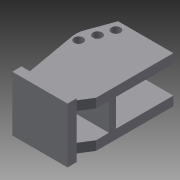
# Autodesk Inventor part: BADAN 3
Saved by Autodesk Inventor 2014 SP2 (Build 180246200, 246)
## iProperties
Created: 2019-06-24
Part Number: BADAN 3
Material: Generic
Document SubType Name: Modeling
Designer: USER PC
Density: 1 g/cm^3
Appearance: Default
Author: USER PC
Autodesk Inventor part; units mm, degrees
ref_plane "YZ Plane" through (0, 0, 0) normal (1, 0, 0) x (0, 1, 0)
ref_plane "XZ Plane" through (0, 0, 0) normal (0, 1, 0) x (-1, 0, 0)
ref_plane "XY Plane" through (0, 0, 0) normal (0, 0, 1) x (1, 0, 0)
sketch "Sketch1" plane through (0, 0, 0) normal (0, 0, 1) x (1, 0, 0)
  line L0 (0, 0) -> (100, 0)
  line L1 (0, 200) -> (150, 200)
  line L2 (150, 200) -> (150, 80)
  line L3 (150, 80) -> (100, 0)
  line L4 (0, 200) -> (-23.9414, 134.2215)
  line L5 (0, 200) -> (70, 200) construction
  line L6 (-23.9414, 134.2215) -> (0, 0)
  constraints: 14 end point, 2 horizontal, 1 equal length, 1 perpendicular
extrude "Extrusion1" add sketch "Sketch1" along normal blind 120
fillet "Fillet1" radius 50 1 edges at (-23.9414, 134.2215, 60)
sketch "Sketch3" plane through (0, 0, 120) normal (0, 0, 1) x (1, 0, 0)
  line L0 (0, 200) -> (-19.341, 146.861) projected
  circle A0 centre (14.3344, 180.9074) radius 10
  line L1 (14.3344, 180.9074) -> (10.9142, 171.5105)
  line L2 (14.3344, 180.9074) -> (133.919, 180.9074) construction
  circle A1 centre (3.6348, 151.5105) radius 10
  circle A2 centre (-7.2843, 121.5105) radius 10
  dimension "d9" = 20
  dimension "d10" = 20
  dimension "d12" = 20
  dimension "d13" = 20
  dimension "d14" = 30
  dimension "d15" = 20
  constraints: 4 end point, 2 centre point, 2 point on line, 1 horizontal, 3 other
  measures "d10" distance from line of L1.start L0
  measures "d12" diameter of A1
  measures "d13" diameter of A2
  measures "d14" vertical distance of A1.centre A2.centre
  measures "d15" vertical distance of A1.centre L1.end
extrude "Extrusion2" cut sketch "Sketch3" against normal blind 120
sketch "Sketch4" plane through (0, 0, 0) normal (1, 0, 0) x (0, 1, 0)
  line L0 (0, 0) -> (200, 0)
  line L1 (200, 100) -> (0, 100)
  line L2 (200, 20) -> (0, 80) construction
  line L3 (0, 20) -> (200, 80) construction
  line L4 (200, 0) -> (200, 20)
  line L5 (200, 80) -> (200, 100)
  line L6 (0, 100) -> (0, 80)
  line L7 (0, 20) -> (0, 0)
  line L8 (60, 50) -> (60, 20)
  line L9 (60, 50) -> (60, 80)
  line L10 (75, 80) -> (75, 20)
  line L11 (200, 20) -> (75, 20)
  line L12 (60, 20) -> (0, 20)
  line L13 (0, 80) -> (60, 80)
  line L14 (75, 80) -> (200, 80)
  point P0 (100, 50)
  constraints: 30 end point, 9 parallel, 6 perpendicular, 3 horizontal, 2 midpoint, 1 collinear
extrude "Extrusion3" cut sketch "Sketch4" along normal mid plane 240 keep common part
sketch "Sketch5" plane through (0, 0, 0) normal (0, 1, 0) x (-1, 0, 0)
  line L0 (10, 110) -> (-110, 110)
  line L1 (-110, 110) -> (-110, -10)
  line L2 (-110, -10) -> (10, -10)
  line L3 (10, -10) -> (10, 110)
  line L4 (10, 110) -> (-110, -10) construction
  line L5 (-110, 110) -> (10, -10) construction
  point P0 (0, 0)
  dimension "d28" = 120
  dimension "d29" = 120
  constraints: 12 end point, 2 parallel, 1 horizontal, 1 perpendicular
  measures "d28" distance of L2.end L1.end
  measures "d29" distance of L1.end L0.end
extrude "Extrusion4" add sketch "Sketch5" against normal blind 20
body "Solid1"
